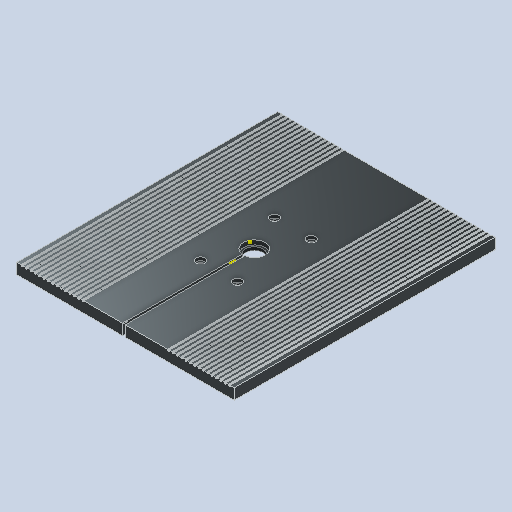
# Autodesk Inventor part: Table_MU
Saved by Autodesk Inventor 2025.2 (Build 292293000, 293)
## iProperties
Created: 2025-05-24
Part Number: Table_MU
Material: Iron, Cast
Document SubType Name: Modeling
Designer: Musa Gamal
Density: 7.15 g/cm^3
Appearance: Iron Gray
Author: Musa Gamal
Autodesk Inventor part; units mm, degrees
ref_plane "YZ Plane" through (0, 0, 0) normal (1, 0, 0) x (0, 1, 0)
ref_plane "XZ Plane" through (0, 0, 0) normal (0, 1, 0) x (-1, 0, 0)
ref_plane "XY Plane" through (0, 0, 0) normal (0, 0, 1) x (1, 0, 0)
sketch "Sketch1" plane through (0, 0, 0) normal (0, 1, 0) x (-1, 0, 0)
  line L0 (455.9236, 615.8581) -> (-544.0764, 615.8581)
  line L1 (-544.0764, 615.8581) -> (-544.0764, -584.1419)
  line L2 (-544.0764, -584.1419) -> (455.9236, -584.1419)
  line L3 (455.9236, -584.1419) -> (455.9236, 615.8581)
  circle A0 centre (-36.0764, 15.8581) radius 50
  line L4 (-36.0764, 15.8581) -> (-30.0764, 15.8581)
  line L5 (-30.0764, 15.8581) -> (-42.0764, 15.8581)
  line L6 (-42.0764, 15.8581) -> (-42.0764, 615.8581)
  line L7 (-42.0764, 15.8581) -> (557.9236, 15.8581) construction
  line L8 (-30.0764, 15.8581) -> (-30.0764, 615.8581)
  line L9 (-30.0764, 15.8581) -> (569.9236, 15.8581) construction
  line L10 (-43.0764, 595.8581) -> (-43.0764, 615.8581)
  line L11 (-29.0764, 595.8581) -> (-29.0764, 615.8581)
  arc A1 (-43.0764, 595.8581) -> (-29.0764, 595.8581) centre (-36.0764, 595.8581) ccw
  point P0 (0, 0)
  point P1 (-8.3732, 8.1039)
  point P2 (-30.0764, 615.8581)
  point P3 (-30.0764, 65.4968)
  point P4 (-42.0764, 65.4968)
  point P5 (-42.0764, 615.8581)
  point P6 (-30.0764, 592.2526)
  point P7 (-42.0764, 592.2526)
  dimension "d0" = 1000
  dimension "d1" = 1200
  dimension "d2" = 100
  dimension "d3" = 600
  dimension "d4" = 12
  dimension "d5" = 6
  dimension "d6" = 20
  dimension "d7" = 6
  dimension "d12" = 492
  constraints: 24 end point, 7 perpendicular, 4 horizontal, 3 point on line, 2 centre point, 2 parallel, 2 point on circle, 1 coincident, 1 tangent
  measures "d0" distance of L3.start L1.end
  measures "d1" distance of L1.end L1.start
  measures "d2" diameter of A0
  measures "d3" distance of L6.start L6.end
  measures "d4" distance between parallel lines of L8 L6
  measures "d5" distance from line of L6 point (-36.076, 15.858)
  measures "d6" distance from line of L0 A1.centre
  measures "d7" distance from line of L8 A1.centre
  measures "d12" distance from line of L3 point (-36.076, 15.858)
extrude "Extrusion1" add sketch "Sketch1" against normal blind 50 contours L3 L2 L1 L0 L10 A1 L6 A0 L8 L11 | L11 A1 L8 L0 | L6 A1 L10 L0
extrude "Extrusion2" cut sketch "Sketch1" against normal blind 5 contours L11 A1 L8 L0 | L6 A1 L10 L0
sketch "Vac" plane through (0, -50, 0) normal (0, -1, 0) x (1, 0, 0)
  arc A0 (30.0764, 65.4968) -> (42.0764, 65.4968) centre (36.0764, 15.8581) ccw projected
  arc A1 (30.0764, 65.4968) -> (42.0764, 65.4968) centre (36.0764, 15.8581) ccw
  circle A2 centre (36.0764, 15.8581) radius 40
  line L0 (42.0764, 65.4968) -> (42.0764, 592.2526) projected
  line L1 (42.0764, 65.4968) -> (42.0764, 55.4056)
  line L2 (30.0764, 65.4968) -> (30.0764, 55.4056)
  point P0 (0, 0)
  point P1 (48.0764, 65.6979)
  point P2 (40.0764, 65.6979)
  dimension "d57" = 80
  constraints: 4 end point, 4 point on circle, 2 centre point, 2 coincident, 1 collinear, 1 concentric, 1 parallel
  measures "d57" diameter of A2
sketch "Bolts" plane through (0, 0, 0) normal (0, 1, 0) x (1, 0, 0)
  circle A0 centre (121.0764, 154.1419) radius 20
  arc A1 (42.0764, -65.4968) -> (30.0764, -65.4968) centre (36.0764, -15.8581) ccw projected
  circle A2 centre (121.0764, 154.1419) radius 10
  line L0 (36.0764, -15.8581) -> (36.0764, 72.4158)
  circle A3 centre (-48.9236, 154.1419) radius 20
  circle A4 centre (-48.9236, 154.1419) radius 10
  line L1 (36.0764, -15.8581) -> (70.1101, -15.8581)
  circle A5 centre (121.0764, -185.8581) radius 20
  circle A6 centre (121.0764, -185.8581) radius 10
  circle A7 centre (-48.9236, -185.8581) radius 20
  circle A8 centre (-48.9236, -185.8581) radius 10
  point P0 (0, 0)
  dimension "d14" = 85
  dimension "d15" = 170
  dimension "d16" = 20
  dimension "d17" = 40
  dimension "d66" = 170
  dimension "d67" = 170
  dimension "d68" = 340
  constraints: 8 centre point, 6 symmetric about line, 5 coincident, 4 end point, 1 horizontal, 1 vertical, 6 other
  measures "d14" horizontal distance of L0.start A0.centre
  measures "d15" vertical distance of L0.start A0.centre
  measures "d16" diameter of A2
  measures "d17" diameter of A0
  measures "d66" distance of A3.centre A0.centre
  measures "d67" vertical distance of L0.start A3.centre
  measures "d68" distance of A0.centre A5.centre
extrude "Extrusion3" cut sketch "Bolts" against normal blind 15 contours A0
extrude "Extrusion4" cut sketch "Bolts" against normal through all contours A2
sketch "Sketch4" plane through (42.0764, -50, 615.8581) normal (0, 0, 1) x (1, 0, 0)
  line L0 (1, 50) -> (1, 45) projected
  line L1 (1, 45) -> (0, 45) projected
  line L2 (0, 45) -> (0, 0) projected
  line L3 (502, 0) -> (0, 0) projected
  line L4 (502, 50) -> (502, 0) projected
  line L5 (1, 50) -> (502, 50) projected
  line L6 (482, 49) -> (482, 45)
  line L7 (481, 44) -> (477, 44)
  line L8 (476, 45) -> (476, 49)
  line L9 (1, 50) -> (502, 50) projected
  line L10 (502, 50) -> (483, 50)
  arc A0 (481, 44) -> (482, 45) centre (481, 45) ccw
  arc A1 (476, 45) -> (477, 44) centre (477, 45) ccw
  arc A2 (483, 50) -> (482, 49) centre (483, 49) ccw
  line L11 (475, 50) -> (447.7677, 50)
  arc A3 (476, 49) -> (475, 50) centre (475, 49) ccw
  arc A4 (463, 50) -> (462, 49) centre (463, 49) ccw
  line L12 (462, 49) -> (462, 45)
  arc A5 (461, 44) -> (462, 45) centre (461, 45) ccw
  line L13 (461, 44) -> (457, 44)
  arc A6 (456, 45) -> (457, 44) centre (457, 45) ccw
  line L14 (456, 45) -> (456, 49)
  arc A7 (456, 49) -> (455, 50) centre (455, 49) ccw
  arc A8 (443, 50) -> (442, 49) centre (443, 49) ccw
  line L15 (442, 49) -> (442, 45)
  arc A9 (441, 44) -> (442, 45) centre (441, 45) ccw
  line L16 (441, 44) -> (437, 44)
  arc A10 (436, 45) -> (437, 44) centre (437, 45) ccw
  line L17 (436, 45) -> (436, 49)
  arc A11 (436, 49) -> (435, 50) centre (435, 49) ccw
  arc A12 (423, 50) -> (422, 49) centre (423, 49) ccw
  line L18 (422, 49) -> (422, 45)
  arc A13 (421, 44) -> (422, 45) centre (421, 45) ccw
  line L19 (421, 44) -> (417, 44)
  arc A14 (416, 45) -> (417, 44) centre (417, 45) ccw
  line L20 (416, 45) -> (416, 49)
  arc A15 (416, 49) -> (415, 50) centre (415, 49) ccw
  arc A16 (403, 50) -> (402, 49) centre (403, 49) ccw
  line L21 (402, 49) -> (402, 45)
  arc A17 (401, 44) -> (402, 45) centre (401, 45) ccw
  line L22 (401, 44) -> (397, 44)
  arc A18 (396, 45) -> (397, 44) centre (397, 45) ccw
  line L23 (396, 45) -> (396, 49)
  arc A19 (396, 49) -> (395, 50) centre (395, 49) ccw
  arc A20 (383, 50) -> (382, 49) centre (383, 49) ccw
  line L24 (382, 49) -> (382, 45)
  arc A21 (381, 44) -> (382, 45) centre (381, 45) ccw
  line L25 (381, 44) -> (377, 44)
  arc A22 (376, 45) -> (377, 44) centre (377, 45) ccw
  line L26 (376, 45) -> (376, 49)
  arc A23 (376, 49) -> (375, 50) centre (375, 49) ccw
  arc A24 (363, 50) -> (362, 49) centre (363, 49) ccw
  line L27 (362, 49) -> (362, 45)
  arc A25 (361, 44) -> (362, 45) centre (361, 45) ccw
  line L28 (361, 44) -> (357, 44)
  arc A26 (356, 45) -> (357, 44) centre (357, 45) ccw
  line L29 (356, 45) -> (356, 49)
  arc A27 (356, 49) -> (355, 50) centre (355, 49) ccw
  arc A28 (343, 50) -> (342, 49) centre (343, 49) ccw
  line L30 (342, 49) -> (342, 45)
  arc A29 (341, 44) -> (342, 45) centre (341, 45) ccw
  line L31 (341, 44) -> (337, 44)
  arc A30 (336, 45) -> (337, 44) centre (337, 45) ccw
  line L32 (336, 45) -> (336, 49)
  arc A31 (336, 49) -> (335, 50) centre (335, 49) ccw
  arc A32 (323, 50) -> (322, 49) centre (323, 49) ccw
  line L33 (322, 49) -> (322, 45)
  arc A33 (321, 44) -> (322, 45) centre (321, 45) ccw
  line L34 (321, 44) -> (317, 44)
  arc A34 (316, 45) -> (317, 44) centre (317, 45) ccw
  line L35 (316, 45) -> (316, 49)
  arc A35 (316, 49) -> (315, 50) centre (315, 49) ccw
  arc A36 (303, 50) -> (302, 49) centre (303, 49) ccw
  line L36 (302, 49) -> (302, 45)
  arc A37 (301, 44) -> (302, 45) centre (301, 45) ccw
  line L37 (301, 44) -> (297, 44)
  arc A38 (296, 45) -> (297, 44) centre (297, 45) ccw
  line L38 (296, 45) -> (296, 49)
  arc A39 (296, 49) -> (295, 50) centre (295, 49) ccw
  arc A40 (283, 50) -> (282, 49) centre (283, 49) ccw
  line L39 (282, 49) -> (282, 45)
  arc A41 (281, 44) -> (282, 45) centre (281, 45) ccw
  line L40 (281, 44) -> (277, 44)
  arc A42 (276, 45) -> (277, 44) centre (277, 45) ccw
  line L41 (276, 45) -> (276, 49)
  arc A43 (276, 49) -> (275, 50) centre (275, 49) ccw
  arc A44 (263, 50) -> (262, 49) centre (263, 49) ccw
  line L42 (262, 49) -> (262, 45)
  arc A45 (261, 44) -> (262, 45) centre (261, 45) ccw
  line L43 (261, 44) -> (257, 44)
  arc A46 (256, 45) -> (257, 44) centre (257, 45) ccw
  line L44 (256, 45) -> (256, 49)
  arc A47 (256, 49) -> (255, 50) centre (255, 49) ccw
  arc A48 (243, 50) -> (242, 49) centre (243, 49) ccw
  line L45 (242, 49) -> (242, 45)
  arc A49 (241, 44) -> (242, 45) centre (241, 45) ccw
  line L46 (241, 44) -> (237, 44)
  arc A50 (236, 45) -> (237, 44) centre (237, 45) ccw
  line L47 (236, 45) -> (236, 49)
  arc A51 (236, 49) -> (235, 50) centre (235, 49) ccw
  arc A52 (223, 50) -> (222, 49) centre (223, 49) ccw
  line L48 (222, 49) -> (222, 45)
  arc A53 (221, 44) -> (222, 45) centre (221, 45) ccw
  line L49 (221, 44) -> (217, 44)
  arc A54 (216, 45) -> (217, 44) centre (217, 45) ccw
  line L50 (216, 45) -> (216, 49)
  arc A55 (216, 49) -> (215, 50) centre (215, 49) ccw
  arc A56 (203, 50) -> (202, 49) centre (203, 49) ccw
  line L51 (202, 49) -> (202, 45)
  arc A57 (201, 44) -> (202, 45) centre (201, 45) ccw
  line L52 (201, 44) -> (197, 44)
  arc A58 (196, 45) -> (197, 44) centre (197, 45) ccw
  line L53 (196, 45) -> (196, 49)
  arc A59 (196, 49) -> (195, 50) centre (195, 49) ccw
  point P0 (-42.0764, 50)
  point P1 (482, 50)
  point P2 (482, 44)
  point P3 (476, 44)
  point P4 (476, 50)
  point P5 (462, 44)
  point P6 (462, 50)
  point P7 (456, 44)
  point P8 (456, 50)
  point P9 (442, 44)
  point P10 (442, 50)
  point P11 (436, 44)
  point P12 (436, 50)
  point P13 (422, 44)
  point P14 (422, 50)
  point P15 (416, 44)
  point P16 (416, 50)
  point P17 (402, 44)
  point P18 (402, 50)
  point P19 (396, 44)
  point P20 (396, 50)
  point P21 (382, 44)
  point P22 (382, 50)
  point P23 (376, 44)
  point P24 (376, 50)
  point P25 (362, 44)
  point P26 (362, 50)
  point P27 (356, 44)
  point P28 (356, 50)
  point P29 (342, 44)
  point P30 (342, 50)
  point P31 (336, 44)
  point P32 (336, 50)
  point P33 (322, 44)
  point P34 (322, 50)
  point P35 (316, 44)
  point P36 (316, 50)
  point P37 (302, 44)
  point P38 (302, 50)
  point P39 (296, 44)
  point P40 (296, 50)
  point P41 (282, 44)
  point P42 (282, 50)
  point P43 (276, 44)
  point P44 (276, 50)
  point P45 (262, 44)
  point P46 (262, 50)
  point P47 (256, 44)
  point P48 (256, 50)
  point P49 (242, 44)
  point P50 (242, 50)
  point P51 (236, 44)
  point P52 (236, 50)
  point P53 (222, 44)
  point P54 (222, 50)
  point P55 (216, 44)
  point P56 (216, 50)
  point P57 (202, 44)
  point P58 (202, 50)
  point P59 (196, 44)
  point P60 (196, 50)
  point P61 (203, 50)
  point P62 (195, 50)
  point P63 (223, 50)
  point P64 (215, 50)
  point P65 (243, 50)
  point P66 (235, 50)
  point P67 (263, 50)
  point P68 (255, 50)
  point P69 (283, 50)
  point P70 (275, 50)
  point P71 (303, 50)
  point P72 (295, 50)
  point P73 (323, 50)
  point P74 (315, 50)
  point P75 (343, 50)
  point P76 (335, 50)
  point P77 (363, 50)
  point P78 (355, 50)
  point P79 (383, 50)
  point P80 (375, 50)
  point P81 (403, 50)
  point P82 (395, 50)
  point P83 (423, 50)
  point P84 (415, 50)
  point P85 (443, 50)
  point P86 (435, 50)
  point P87 (463, 50)
  point P88 (455, 50)
  point P89 (483, 50)
  point P90 (475, 50)
  dimension "d26" = 6
  dimension "d27" = 6
  dimension "d28" = 6
  dimension "d29" = 1
  dimension "d30" = 1
  dimension "d31" = 1
  dimension "d32" = 1
  dimension "d33" = 20
  dimension "d36" = 20
  constraints: 224 horizontal alignment, 120 point on circle, 94 end point, 93 point on line, 60 centre point, 56 equal radius, 28 parallel, 14 collinear, 8 tangent, 1 horizontal, 1 perpendicular, 1 vertical, 3 other
  measures "d26" distance of point (482, 50) point (482, 44)
  measures "d27" distance of point (482, 44) point (476, 44)
  measures "d28" distance of point (476, 44) point (476, 50)
  measures "d29" radius of A0
  measures "d30" radius of A1
  measures "d31" radius of A2
  measures "d32" radius of A3
  measures "d33" distance between parallel lines of L4 L6
  measures "d36" distance of A2.centre A4.centre
extrude "Extrusion5" cut sketch "Sketch4" against normal through all contours L5 A56 L51 A57 L52 A58 L53 A59 | L5 A52 L48 A53 L49 A54 L50 A55 | L5 A48 L45 A49 L46 A50 L47 A51 | A2 L6 A0 L7 A1 L8 A3 L5 | L5 A44 L42 A45 L43 A46 L44 A47 | A4 L12 A5 L13 A6 L14 A7 L5 | L5 A40 L39 A41 L40 A42 L41 A43 | A8 L15 A9 L16 A10 L17 A11 L5 | L5 A36 L36 A37 L37 A38 L38 A39 | A12 L18 A13 L19 A14 L20 A15 L5 | L5 A32 L33 A33 L34 A34 L35 A35 | A16 L21 A17 L22 A18 L23 A19 L5 | L5 A28 L30 A29 L31 A30 L32 A31 | A20 L24 A21 L25 A22 L26 A23 L5 | L5 A24 L27 A25 L28 A26 L29 A27
sketch "Sketch5" plane through (-455.9236, -50, 615.8581) normal (0, 0, 1) x (1, 0, 0)
  line L0 (0, 50) -> (485, 50) projected
  line L1 (0, 50) -> (19, 50)
  line L2 (20, 49) -> (20, 45)
  line L3 (21, 44) -> (25, 44)
  line L4 (26, 45) -> (26, 49)
  arc A0 (20, 45) -> (21, 44) centre (21, 45) ccw
  arc A1 (25, 44) -> (26, 45) centre (25, 45) ccw
  arc A2 (20, 49) -> (19, 50) centre (19, 49) ccw
  line L5 (27, 50) -> (24.777, 50)
  arc A3 (27, 50) -> (26, 49) centre (27, 49) ccw
  line L6 (0, 50) -> (0, 0) projected
  arc A4 (47, 50) -> (46, 49) centre (47, 49) ccw
  line L7 (46, 45) -> (46, 49)
  arc A5 (45, 44) -> (46, 45) centre (45, 45) ccw
  line L8 (41, 44) -> (45, 44)
  arc A6 (40, 45) -> (41, 44) centre (41, 45) ccw
  line L9 (40, 49) -> (40, 45)
  arc A7 (40, 49) -> (39, 50) centre (39, 49) ccw
  arc A8 (67, 50) -> (66, 49) centre (67, 49) ccw
  line L10 (66, 45) -> (66, 49)
  arc A9 (65, 44) -> (66, 45) centre (65, 45) ccw
  line L11 (61, 44) -> (65, 44)
  arc A10 (60, 45) -> (61, 44) centre (61, 45) ccw
  line L12 (60, 49) -> (60, 45)
  arc A11 (60, 49) -> (59, 50) centre (59, 49) ccw
  arc A12 (87, 50) -> (86, 49) centre (87, 49) ccw
  line L13 (86, 45) -> (86, 49)
  arc A13 (85, 44) -> (86, 45) centre (85, 45) ccw
  line L14 (81, 44) -> (85, 44)
  arc A14 (80, 45) -> (81, 44) centre (81, 45) ccw
  line L15 (80, 49) -> (80, 45)
  arc A15 (80, 49) -> (79, 50) centre (79, 49) ccw
  arc A16 (107, 50) -> (106, 49) centre (107, 49) ccw
  line L16 (106, 45) -> (106, 49)
  arc A17 (105, 44) -> (106, 45) centre (105, 45) ccw
  line L17 (101, 44) -> (105, 44)
  arc A18 (100, 45) -> (101, 44) centre (101, 45) ccw
  line L18 (100, 49) -> (100, 45)
  arc A19 (100, 49) -> (99, 50) centre (99, 49) ccw
  arc A20 (127, 50) -> (126, 49) centre (127, 49) ccw
  line L19 (126, 45) -> (126, 49)
  arc A21 (125, 44) -> (126, 45) centre (125, 45) ccw
  line L20 (121, 44) -> (125, 44)
  arc A22 (120, 45) -> (121, 44) centre (121, 45) ccw
  line L21 (120, 49) -> (120, 45)
  arc A23 (120, 49) -> (119, 50) centre (119, 49) ccw
  arc A24 (147, 50) -> (146, 49) centre (147, 49) ccw
  line L22 (146, 45) -> (146, 49)
  arc A25 (145, 44) -> (146, 45) centre (145, 45) ccw
  line L23 (141, 44) -> (145, 44)
  arc A26 (140, 45) -> (141, 44) centre (141, 45) ccw
  line L24 (140, 49) -> (140, 45)
  arc A27 (140, 49) -> (139, 50) centre (139, 49) ccw
  arc A28 (167, 50) -> (166, 49) centre (167, 49) ccw
  line L25 (166, 45) -> (166, 49)
  arc A29 (165, 44) -> (166, 45) centre (165, 45) ccw
  line L26 (161, 44) -> (165, 44)
  arc A30 (160, 45) -> (161, 44) centre (161, 45) ccw
  line L27 (160, 49) -> (160, 45)
  arc A31 (160, 49) -> (159, 50) centre (159, 49) ccw
  arc A32 (187, 50) -> (186, 49) centre (187, 49) ccw
  line L28 (186, 45) -> (186, 49)
  arc A33 (185, 44) -> (186, 45) centre (185, 45) ccw
  line L29 (181, 44) -> (185, 44)
  arc A34 (180, 45) -> (181, 44) centre (181, 45) ccw
  line L30 (180, 49) -> (180, 45)
  arc A35 (180, 49) -> (179, 50) centre (179, 49) ccw
  arc A36 (207, 50) -> (206, 49) centre (207, 49) ccw
  line L31 (206, 45) -> (206, 49)
  arc A37 (205, 44) -> (206, 45) centre (205, 45) ccw
  line L32 (201, 44) -> (205, 44)
  arc A38 (200, 45) -> (201, 44) centre (201, 45) ccw
  line L33 (200, 49) -> (200, 45)
  arc A39 (200, 49) -> (199, 50) centre (199, 49) ccw
  arc A40 (227, 50) -> (226, 49) centre (227, 49) ccw
  line L34 (226, 45) -> (226, 49)
  arc A41 (225, 44) -> (226, 45) centre (225, 45) ccw
  line L35 (221, 44) -> (225, 44)
  arc A42 (220, 45) -> (221, 44) centre (221, 45) ccw
  line L36 (220, 49) -> (220, 45)
  arc A43 (220, 49) -> (219, 50) centre (219, 49) ccw
  arc A44 (247, 50) -> (246, 49) centre (247, 49) ccw
  line L37 (246, 45) -> (246, 49)
  arc A45 (245, 44) -> (246, 45) centre (245, 45) ccw
  line L38 (241, 44) -> (245, 44)
  arc A46 (240, 45) -> (241, 44) centre (241, 45) ccw
  line L39 (240, 49) -> (240, 45)
  arc A47 (240, 49) -> (239, 50) centre (239, 49) ccw
  arc A48 (267, 50) -> (266, 49) centre (267, 49) ccw
  line L40 (266, 45) -> (266, 49)
  arc A49 (265, 44) -> (266, 45) centre (265, 45) ccw
  line L41 (261, 44) -> (265, 44)
  arc A50 (260, 45) -> (261, 44) centre (261, 45) ccw
  line L42 (260, 49) -> (260, 45)
  arc A51 (260, 49) -> (259, 50) centre (259, 49) ccw
  arc A52 (287, 50) -> (286, 49) centre (287, 49) ccw
  line L43 (286, 45) -> (286, 49)
  arc A53 (285, 44) -> (286, 45) centre (285, 45) ccw
  line L44 (281, 44) -> (285, 44)
  arc A54 (280, 45) -> (281, 44) centre (281, 45) ccw
  line L45 (280, 49) -> (280, 45)
  arc A55 (280, 49) -> (279, 50) centre (279, 49) ccw
  arc A56 (307, 50) -> (306, 49) centre (307, 49) ccw
  line L46 (306, 45) -> (306, 49)
  arc A57 (305, 44) -> (306, 45) centre (305, 45) ccw
  line L47 (301, 44) -> (305, 44)
  arc A58 (300, 45) -> (301, 44) centre (301, 45) ccw
  line L48 (300, 49) -> (300, 45)
  arc A59 (300, 49) -> (299, 50) centre (299, 49) ccw
  point P0 (455.9236, 50)
  point P1 (120.0321, 50)
  point P2 (20, 50)
  point P3 (20, 44)
  point P4 (26, 44)
  point P5 (26, 50)
  point P6 (46, 44)
  point P7 (46, 50)
  point P8 (40, 44)
  point P9 (40, 50)
  point P10 (66, 44)
  point P11 (66, 50)
  point P12 (60, 44)
  point P13 (60, 50)
  point P14 (86, 44)
  point P15 (86, 50)
  point P16 (80, 44)
  point P17 (80, 50)
  point P18 (106, 44)
  point P19 (106, 50)
  point P20 (100, 44)
  point P21 (100, 50)
  point P22 (126, 44)
  point P23 (126, 50)
  point P24 (120, 44)
  point P25 (120, 50)
  point P26 (146, 44)
  point P27 (146, 50)
  point P28 (140, 44)
  point P29 (140, 50)
  point P30 (166, 44)
  point P31 (166, 50)
  point P32 (160, 44)
  point P33 (160, 50)
  point P34 (186, 44)
  point P35 (186, 50)
  point P36 (180, 44)
  point P37 (180, 50)
  point P38 (206, 44)
  point P39 (206, 50)
  point P40 (200, 44)
  point P41 (200, 50)
  point P42 (226, 44)
  point P43 (226, 50)
  point P44 (220, 44)
  point P45 (220, 50)
  point P46 (246, 44)
  point P47 (246, 50)
  point P48 (240, 44)
  point P49 (240, 50)
  point P50 (266, 44)
  point P51 (266, 50)
  point P52 (260, 44)
  point P53 (260, 50)
  point P54 (286, 44)
  point P55 (286, 50)
  point P56 (280, 44)
  point P57 (280, 50)
  point P58 (306, 44)
  point P59 (306, 50)
  point P60 (300, 44)
  point P61 (300, 50)
  point P62 (27, 50)
  point P63 (19, 50)
  point P64 (47, 50)
  point P65 (39, 50)
  point P66 (67, 50)
  point P67 (59, 50)
  point P68 (87, 50)
  point P69 (79, 50)
  point P70 (107, 50)
  point P71 (99, 50)
  point P72 (127, 50)
  point P73 (119, 50)
  point P74 (139, 50)
  point P75 (159, 50)
  point P76 (179, 50)
  point P77 (199, 50)
  point P78 (219, 50)
  point P79 (239, 50)
  point P80 (259, 50)
  point P81 (279, 50)
  point P82 (299, 50)
  dimension "d43" = 6
  dimension "d44" = 6
  dimension "d45" = 1
  dimension "d46" = 1
  dimension "d47" = 20
  dimension "d50" = 20
  constraints: 224 horizontal alignment, 120 point on circle, 94 end point, 94 point on line, 60 centre point, 58 equal radius, 28 parallel, 14 collinear, 8 tangent, 3 perpendicular, 3 other
  measures "d43" distance of point (20, 50) point (20, 44)
  measures "d44" distance of point (20, 44) point (26, 44)
  measures "d45" radius of A0
  measures "d46" radius of A3
  measures "d47" distance between parallel lines of L6 L2
  measures "d50" distance of A3.centre A4.centre
extrude "Extrusion6" cut sketch "Sketch5" against normal through all
extrude "Extrusion7" add sketch "Vac" against normal blind 30 contours L2 A2 L1 A0
extrude "Extrusion8" cut sketch "Bolts" against normal blind 15 contours A3 | A5 | A7
sketch "Sketch7" plane through (0, -50, 0) normal (0, -1, 0) x (1, 0, 0)
  arc A0 (30.0764, 55.4056) -> (42.0764, 55.4056) centre (36.0764, 15.8581) ccw projected
  arc A1 (30.0764, 55.4056) -> (42.0764, 55.4056) centre (36.0764, 15.8581) ccw
  line L0 (42.0764, 55.4056) -> (42.0764, 71.1073)
  line L1 (42.0764, 615.8581) -> (42.0764, 55.4056) projected
  line L2 (30.0764, 55.4056) -> (30.0764, 69.2029)
  line L3 (36.0764, 95.8581) -> (126.0764, 95.8581)
  line L4 (136.0764, 85.8581) -> (136.0764, -54.1419)
  line L5 (126.0764, -64.1419) -> (-53.9236, -64.1419)
  line L6 (-63.9236, -54.1419) -> (-63.9236, 85.8581)
  line L7 (-53.9236, 95.8581) -> (36.0764, 95.8581)
  circle A2 centre (116.0764, -44.1419) radius 5
  circle A3 centre (116.0764, 75.8581) radius 5
  circle A4 centre (-43.9236, 80.1049) radius 5
  circle A5 centre (-43.9236, -39.8951) radius 5
  line L8 (30.0764, 55.4056) -> (30.0764, 615.8581) projected
  arc A6 (126.0764, -64.1419) -> (136.0764, -54.1419) centre (126.0764, -54.1419) ccw
  arc A7 (136.0764, 85.8581) -> (126.0764, 95.8581) centre (126.0764, 85.8581) ccw
  arc A8 (-53.9236, 95.8581) -> (-63.9236, 85.8581) centre (-53.9236, 85.8581) ccw
  arc A9 (-63.9236, -54.1419) -> (-53.9236, -64.1419) centre (-53.9236, -54.1419) ccw
  point P0 (0, 0)
  point P1 (136.0764, 95.8581)
  point P2 (136.0764, -64.1419)
  point P3 (-63.9236, -64.1419)
  point P4 (-63.9236, 95.8581)
  point P5 (42.0764, 95.8581)
  point P6 (30.0764, 95.8581)
  dimension "d71" = 80
  dimension "d73" = 160
  dimension "d74" = 200
  dimension "d75" = 10
  dimension "d76" = 10
  dimension "d77" = 10
  dimension "d78" = 10
  dimension "d79" = 20
  dimension "d80" = 120
  dimension "d81" = 160
  dimension "d82" = 20
  dimension "d83" = 120
  dimension "d84" = 160
  dimension "d86" = 100
  dimension "d91" = 10
  constraints: 14 end point, 10 point on circle, 9 centre point, 9 point on line, 8 tangent, 4 equal radius, 3 perpendicular, 2 horizontal, 1 coincident, 1 vertical
  measures "d71" distance of A1.centre L3.start
  measures "d73" distance of point (136.076, 95.858) point (136.076, -64.142)
  measures "d74" distance of point (136.076, -64.142) point (-63.924, -64.142)
  measures "d75" diameter of A2
  measures "d76" diameter of A3
  measures "d77" diameter of A4
  measures "d78" diameter of A5
  measures "d79" distance from line of A2.centre L5
  measures "d80" distance of A2.centre A3.centre
  measures "d81" horizontal distance of A5.centre A2.centre
  measures "d82" distance from line of A2.centre L4
  measures "d83" distance of A5.centre A4.centre
  measures "d84" horizontal distance of A3.centre A4.centre
  measures "d86" distance from line of L6 A0.centre
  measures "d91" radius of A6
extrude "Extrusion9" cut sketch "Bolts" against normal through all contours A4 | A6 | A8
extrude "Extrusion10" cut sketch "Sketch7" against normal blind 15
extrude "Extrusion11" cut sketch "Sketch7" against normal blind 25 contours A2 | A3 | A4 | A5
sketch "Sketch8" plane through (0, 0, 0) normal (0, 1, 0) x (1, 0, 0)
  line L0 (39.0278, -131.1774) -> (37.7778, -131.1774) projected
  line L1 (37.7778, -131.1774) -> (37.8475, -105.1967) projected
  line L2 (39.0975, -105.1967) -> (39.0278, -131.1774) projected
  point P0 (0, 0)
sketch "Sketch9" plane through (0, -50, 0) normal (0, -1, 0) x (1, 0, 0)
  arc A0 (119.7585, 182.228) -> (137.7585, 180.8962) centre (129.0764, 185.8581) ccw projected
  spline S0 degree 3 poles (137.7585, 190.82) (138.0235, 190.3563) (138.2544, 189.8653) (138.8686, 188.2217) (139.0764, 187.0006) (139.0764, 184.7157) (138.8686, 183.4946) (138.2544, 181.851) (138.0235, 181.3599) (137.7585, 180.8962) knots 4.168299 4.168299 4.168299 4.168299 4.321059 4.321059 4.663784 4.663784 5.006509 5.006509 5.15927 5.15927 5.15927 5.15927 projected
  arc A1 (137.7585, 190.82) -> (119.7585, 189.4882) centre (129.0764, 185.8581) ccw projected
  spline S1 degree 3 poles (119.7585, 182.228) (119.7182, 182.3314) (119.6796, 182.4356) (119.2615, 183.6246) (119.0764, 184.7812) (119.0764, 186.9351) (119.2615, 188.0917) (119.6796, 189.2807) (119.7182, 189.3848) (119.7585, 189.4882) knots 4.143007 4.143007 4.143007 4.143007 4.17424 4.17424 4.497329 4.497329 4.820418 4.820418 4.851651 4.851651 4.851651 4.851651 projected
  spline S2 degree 3 poles (-32.2415, 190.82) (-31.9765, 190.3563) (-31.7456, 189.8653) (-31.1314, 188.2217) (-30.9236, 187.0006) (-30.9236, 184.7157) (-31.1314, 183.4946) (-31.7456, 181.851) (-31.9765, 181.3599) (-32.2415, 180.8962) knots 4.168299 4.168299 4.168299 4.168299 4.321059 4.321059 4.663784 4.663784 5.006509 5.006509 5.15927 5.15927 5.15927 5.15927 projected
  arc A2 (-50.2415, 182.228) -> (-32.2415, 180.8962) centre (-40.9236, 185.8581) ccw projected
  spline S3 degree 3 poles (-50.2415, 182.228) (-50.2818, 182.3314) (-50.3204, 182.4356) (-50.7385, 183.6246) (-50.9236, 184.7812) (-50.9236, 186.9351) (-50.7385, 188.0917) (-50.3204, 189.2807) (-50.2818, 189.3848) (-50.2415, 189.4882) knots 4.143007 4.143007 4.143007 4.143007 4.17424 4.17424 4.497329 4.497329 4.820418 4.820418 4.851651 4.851651 4.851651 4.851651 projected
  arc A3 (-32.2415, 190.82) -> (-50.2415, 189.4882) centre (-40.9236, 185.8581) ccw projected
  arc A4 (-50.2415, -157.772) -> (-32.2415, -159.1038) centre (-40.9236, -154.1419) ccw projected
  spline S4 degree 3 poles (-32.2415, -149.18) (-31.9765, -149.6437) (-31.7456, -150.1347) (-31.1314, -151.7783) (-30.9236, -152.9994) (-30.9236, -155.2843) (-31.1314, -156.5054) (-31.7456, -158.149) (-31.9765, -158.6401) (-32.2415, -159.1038) knots 4.168299 4.168299 4.168299 4.168299 4.321059 4.321059 4.663784 4.663784 5.006509 5.006509 5.15927 5.15927 5.15927 5.15927 projected
  spline S5 degree 3 poles (-50.2415, -157.772) (-50.2818, -157.6686) (-50.3204, -157.5644) (-50.7385, -156.3754) (-50.9236, -155.2188) (-50.9236, -153.0649) (-50.7385, -151.9083) (-50.3204, -150.7193) (-50.2818, -150.6152) (-50.2415, -150.5118) knots 4.143007 4.143007 4.143007 4.143007 4.17424 4.17424 4.497329 4.497329 4.820418 4.820418 4.851651 4.851651 4.851651 4.851651 projected
  arc A5 (-32.2415, -149.18) -> (-50.2415, -150.5118) centre (-40.9236, -154.1419) ccw projected
  arc A6 (119.7585, -157.772) -> (137.7585, -159.1038) centre (129.0764, -154.1419) ccw projected
  spline S6 degree 3 poles (137.7585, -149.18) (138.0235, -149.6437) (138.2544, -150.1347) (138.8686, -151.7783) (139.0764, -152.9994) (139.0764, -155.2843) (138.8686, -156.5054) (138.2544, -158.149) (138.0235, -158.6401) (137.7585, -159.1038) knots 4.168299 4.168299 4.168299 4.168299 4.321059 4.321059 4.663784 4.663784 5.006509 5.006509 5.15927 5.15927 5.15927 5.15927 projected
  arc A7 (137.7585, -149.18) -> (119.7585, -150.5118) centre (129.0764, -154.1419) ccw projected
  spline S7 degree 3 poles (119.7585, -157.772) (119.7182, -157.6686) (119.6796, -157.5644) (119.2615, -156.3754) (119.0764, -155.2188) (119.0764, -153.0649) (119.2615, -151.9083) (119.6796, -150.7193) (119.7182, -150.6152) (119.7585, -150.5118) knots 4.143007 4.143007 4.143007 4.143007 4.17424 4.17424 4.497329 4.497329 4.820418 4.820418 4.851651 4.851651 4.851651 4.851651 projected
  point P0 (0, 0)
sketch "Sketch10" plane through (0, 0, 0) normal (0, 1, 0) x (1, 0, 0)
  circle A0 centre (121.0764, -185.8581) radius 20 projected
  circle A1 centre (-48.9236, -185.8581) radius 20 projected
  circle A2 centre (-48.9236, 154.1419) radius 20 projected
  circle A3 centre (121.0764, 154.1419) radius 20 projected
  point P0 (0, 0)
extrude "Extrusion12" add sketch "Sketch10" against normal up to surface (50 mm away)
extrude "Extrusion13" cut sketch "Sketch9" against normal through all
sketch "Sketch11" plane through (0, 0, 0) normal (0, 1, 0) x (1, 0, 0)
  arc A0 (119.7585, -189.4882) -> (137.7585, -190.82) centre (129.0764, -185.8581) ccw projected
  circle A1 centre (129.0764, -185.8581) radius 20
  arc A2 (-50.2415, -189.4882) -> (-32.2415, -190.82) centre (-40.9236, -185.8581) ccw projected
  circle A3 centre (-40.9236, -185.8581) radius 20
  arc A4 (-50.2415, 150.5118) -> (-32.2415, 149.18) centre (-40.9236, 154.1419) ccw projected
  circle A5 centre (-40.9236, 154.1419) radius 20
  arc A6 (119.7585, 150.5118) -> (137.7585, 149.18) centre (129.0764, 154.1419) ccw projected
  circle A7 centre (129.0764, 154.1419) radius 20
  spline S0 degree 3 poles (-32.2415, -180.8962) (-31.9728, -181.3664) (-31.7423, -181.8585) (-31.3383, -182.9427) (-31.179, -183.5398) (-30.9758, -184.708) (-30.9242, -185.2781) (-30.923, -186.425) (-30.9747, -187.0018) (-31.179, -188.1764) (-31.3383, -188.7735) (-31.7423, -189.8577) (-31.9728, -190.3498) (-32.2415, -190.82) knots 0 0 0 0 0.156468 0.156468 0.334243 0.334243 0.499045 0.499045 0.665756 0.665756 0.843532 0.843532 1 1 1 1 projected
  arc A8 (-32.2415, -180.8962) -> (-50.2415, -182.228) centre (-40.9236, -185.8581) ccw projected
  spline S1 degree 5 poles (-50.2415, -189.4882) (-50.5107, -188.7972) (-50.7148, -188.0806) (-50.8488, -187.3475) (-50.9231, -186.6064) (-50.9242, -185.1212) (-50.8504, -184.3772) (-50.7163, -183.6412) (-50.5117, -182.9217) (-50.2415, -182.228) knots 0 0 0 0 0 0 0.499046 0.499046 0.499046 0.499046 1 1 1 1 1 1 projected
  spline S2 degree 3 poles (137.7585, -180.8962) (138.0272, -181.3664) (138.2577, -181.8585) (138.6617, -182.9427) (138.821, -183.5398) (139.0242, -184.708) (139.0758, -185.2781) (139.077, -186.425) (139.0253, -187.0018) (138.821, -188.1764) (138.6617, -188.7735) (138.2577, -189.8577) (138.0272, -190.3498) (137.7585, -190.82) knots 0 0 0 0 0.156468 0.156468 0.334243 0.334243 0.499045 0.499045 0.665756 0.665756 0.843532 0.843532 1 1 1 1 projected
  arc A9 (137.7585, -180.8962) -> (119.7585, -182.228) centre (129.0764, -185.8581) ccw projected
  spline S3 degree 5 poles (119.7585, -189.4882) (119.4893, -188.7972) (119.2852, -188.0806) (119.1512, -187.3475) (119.0769, -186.6064) (119.0758, -185.1212) (119.1496, -184.3772) (119.2837, -183.6412) (119.4883, -182.9217) (119.7585, -182.228) knots 0 0 0 0 0 0 0.499046 0.499046 0.499046 0.499046 1 1 1 1 1 1 projected
  spline S4 degree 3 poles (137.7585, 159.1038) (138.0272, 158.6336) (138.2577, 158.1415) (138.6617, 157.0573) (138.821, 156.4602) (139.0242, 155.292) (139.0758, 154.7219) (139.077, 153.575) (139.0253, 152.9982) (138.821, 151.8236) (138.6617, 151.2265) (138.2577, 150.1423) (138.0272, 149.6502) (137.7585, 149.18) knots 0 0 0 0 0.156468 0.156468 0.334243 0.334243 0.499045 0.499045 0.665756 0.665756 0.843532 0.843532 1 1 1 1 projected
  arc A10 (137.7585, 159.1038) -> (119.7585, 157.772) centre (129.0764, 154.1419) ccw projected
  spline S5 degree 5 poles (119.7585, 150.5118) (119.4893, 151.2028) (119.2852, 151.9194) (119.1512, 152.6525) (119.0769, 153.3936) (119.0758, 154.8788) (119.1496, 155.6228) (119.2837, 156.3588) (119.4883, 157.0783) (119.7585, 157.772) knots 0 0 0 0 0 0 0.499046 0.499046 0.499046 0.499046 1 1 1 1 1 1 projected
  spline S6 degree 5 poles (-50.2415, 150.5118) (-50.5107, 151.2028) (-50.7148, 151.9194) (-50.8488, 152.6525) (-50.9231, 153.3936) (-50.9242, 154.8788) (-50.8504, 155.6228) (-50.7163, 156.3588) (-50.5117, 157.0783) (-50.2415, 157.772) knots 0 0 0 0 0 0 0.499046 0.499046 0.499046 0.499046 1 1 1 1 1 1 projected
  arc A11 (-32.2415, 159.1038) -> (-50.2415, 157.772) centre (-40.9236, 154.1419) ccw projected
  spline S7 degree 3 poles (-32.2415, 159.1038) (-31.9728, 158.6336) (-31.7423, 158.1415) (-31.3383, 157.0573) (-31.179, 156.4602) (-30.9758, 155.292) (-30.9242, 154.7219) (-30.923, 153.575) (-30.9747, 152.9982) (-31.179, 151.8236) (-31.3383, 151.2265) (-31.7423, 150.1423) (-31.9728, 149.6502) (-32.2415, 149.18) knots 0 0 0 0 0.156468 0.156468 0.334243 0.334243 0.499045 0.499045 0.665756 0.665756 0.843532 0.843532 1 1 1 1 projected
  point P0 (0, 0)
  dimension "d96" = 40
  dimension "d97" = 40
  dimension "d98" = 40
  dimension "d99" = 40
  constraints: 8 vertical alignment, 4 centre point, 4 coincident
  measures "d96" diameter of A1
  measures "d97" diameter of A3
  measures "d98" diameter of A5
  measures "d99" diameter of A7
extrude "Extrusion14" cut sketch "Sketch11" against normal blind 15
equation "\"d2\" = 0.1 * d0"
equation "\"d3\" = 0.5 * d1"
equation "\"d5\" = 0.5 * d4"
equation "\"d7\" = d5"
equation "\"d17\" = 2 * d16"
equation "\"d86\" = 0.5 * d74"
body "Solid1"
